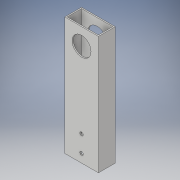
# Autodesk Inventor part: vertical leg
Saved by Autodesk Inventor 2018 (Build 220112000, 112)
## iProperties
Created: 2020-01-24
Part Number: vertical leg
Material: Generic
Document SubType Name: Modeling
Designer: s-2513225
Density: 1 g/cm^3
Appearance: Default
Author: s-2513225
Autodesk Inventor part; units mm, degrees
ref_plane "YZ Plane" through (0, 0, 0) normal (1, 0, 0) x (0, 1, 0)
ref_plane "XZ Plane" through (0, 0, 0) normal (0, 1, 0) x (-1, 0, 0)
ref_plane "XY Plane" through (0, 0, 0) normal (0, 0, 1) x (1, 0, 0)
sketch "Sketch1" plane through (0, 0, 0) normal (0, 0, 1) x (1, 0, 0)
  line L0 (0, 0) -> (50.8, 0)
  line L1 (50.8, 0) -> (50.8, 177.8)
  line L2 (50.8, 177.8) -> (0, 177.8)
  line L3 (0, 177.8) -> (0, 0)
  dimension "d0" = 50.8
  dimension "d1" = 177.8
  constraints: 8 end point, 2 parallel, 1 horizontal, 1 perpendicular
  measures "d0" distance of L2.end L1.end
  measures "d1" distance of L1.end L0.end
extrude "Extrusion1" add sketch "Sketch1" along normal blind 25.4
sketch "Sketch2" plane through (0, 177.8, 0) normal (0, 1, 0) x (1, 0, 0)
  line L0 (0, 0) -> (0, -25.4) projected
  line L1 (50.8, -25.4) -> (0, -25.4) projected
  line L2 (50.8, 0) -> (50.8, -25.4) projected
  line L3 (50.8, 0) -> (0, 0) projected
  line L4 (48.895, -23.495) -> (1.905, -23.495)
  line L5 (1.905, -23.495) -> (1.905, -1.905)
  line L6 (1.905, -1.905) -> (48.895, -1.905)
  line L7 (48.895, -1.905) -> (48.895, -23.495)
  dimension "d4" = 1.905
  constraints: 8 end point, 3 other
  measures "d4" distance between parallel lines of L2 L7
extrude "Extrusion2" cut sketch "Sketch2" against normal blind 508 contours L4 L5 L6 L7
sketch "Sketch3" plane through (0, 0, 25.4) normal (0, 0, 1) x (1, 0, 0)
  line L0 (1.905, 0) -> (48.895, 0) construction
  line L1 (25.4, 0) -> (25.4, 12.7) construction
  line L2 (25.4, 12.7) -> (25.4, 38.1) construction
  line L3 (48.895, 177.8) -> (1.905, 177.8) construction
  line L4 (25.4, 177.8) -> (25.4, 152.4) construction
  circle A0 centre (25.4, 152.4) radius 14.2557
  circle A1 centre (25.4, 12.7) radius 2.5797
  circle A2 centre (25.4, 38.1) radius 2.5797
  point P0 (0, 0)
  dimension "d7" = 12.7
  dimension "d8" = 25.4
  dimension "d9" = 25.4
  dimension "d10" = 28.5115
  dimension "d11" = 5.1594
  dimension "d12" = 5.1594
  constraints: 6 end point, 3 centre point, 3 coincident, 2 midpoint, 2 vertical, 1 point on line
  measures "d7" distance of L1.start L1.end
  measures "d8" distance of L1.end L2.end
  measures "d9" distance of L4.start L4.end
  measures "d10" diameter of A0
  measures "d11" diameter of A1
  measures "d12" diameter of A2
extrude "Extrusion3" cut sketch "Sketch3" against normal blind 508
body "Solid1"
